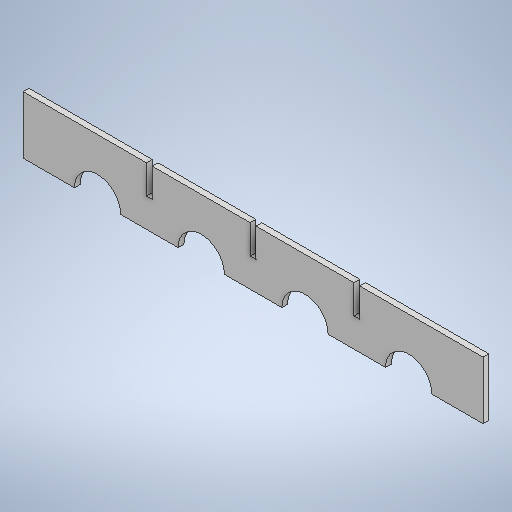
# Autodesk Inventor part: BSH 083 amplifier bottom
Saved by Autodesk Inventor 2025 (Build 290162010, 162A)
## iProperties
Created: 2024-08-04
Part Number: BSH 083 amplifier bottom
Material: Stainless Steel
Document SubType Name: Sheet Metal
Designer: pokla
Density: 8 g/cm^3
Sheet Metal Rule: AISI304 2mm Die16
Appearance: Default
Author: pokla
Autodesk Inventor part; units mm, degrees
ref_plane "YZ Plane" through (0, 0, 0) normal (1, 0, 0) x (0, 1, 0)
ref_plane "XZ Plane" through (0, 0, 0) normal (0, 1, 0) x (-1, 0, 0)
ref_plane "XY Plane" through (0, 0, 0) normal (0, 0, 1) x (1, 0, 0)
sketch "Sketch1" plane through (0, 0, 0) normal (0, 0, 1) x (1, 0, 0)
  circle A0 centre (0, 0) radius 400 construction
  line L0 (-399, 5) -> (399, 5)
  line L1 (399, 5) -> (399, -5)
  line L2 (399, -5) -> (-399, -5)
  line L3 (-399, -5) -> (-399, 5)
  line L4 (-399, 5) -> (399, -5) construction
  dimension "d0" = 800
  dimension "d1" = 10
  dimension "d2" = 798
  constraints: 10 end point, 3 coincident, 2 parallel, 1 centre point, 1 horizontal, 1 midpoint, 1 perpendicular
  measures "d0" diameter of A0
  measures "d1" distance of L0.end L1.end
  measures "d2" distance of L0.start L0.end
extrude "Extrusion1" add sketch "Sketch1" along normal blind 100
sketch "Sketch2" plane through (-399, -5, 0) normal (0, -1, 0) x (1, 0, 0)
  circle A0 centre (309, 0) radius 40
  line L0 (0, 0) -> (798, 0) projected
  circle A1 centre (129, 0) radius 40
  circle A2 centre (489, 0) radius 40
  circle A3 centre (669, 0) radius 40
  line L1 (394, 100) -> (404, 100)
  line L2 (404, 100) -> (404, 50)
  line L3 (404, 50) -> (394, 50)
  line L4 (394, 50) -> (394, 100)
  line L5 (0, 100) -> (798, 100) projected
  line L6 (214, 100) -> (224, 100)
  line L7 (224, 100) -> (224, 50)
  line L8 (224, 50) -> (214, 50)
  line L9 (214, 50) -> (214, 100)
  line L10 (574, 100) -> (584, 100)
  line L11 (584, 100) -> (584, 50)
  line L12 (584, 50) -> (574, 50)
  line L13 (574, 50) -> (574, 100)
  point P0 (399, 0)
  point P1 (399, 0)
  point P2 (399, 0)
  point P3 (399, 0)
  point P4 (399, 100)
  point P5 (219, 100)
  point P6 (399, 100)
  point P7 (399, 100)
  point P8 (579, 100)
  point P9 (399, 100)
  point P10 (399, 100)
  point P11 (709, 0)
  point P12 (629, 0)
  point P13 (529, 0)
  point P14 (449, 0)
  point P15 (269, 0)
  point P16 (349, 0)
  point P17 (169, 0)
  point P18 (89, 0)
  dimension "d5" = 80
  dimension "d7" = 90
  dimension "d8" = 80
  dimension "d9" = 180
  dimension "d10" = 80
  dimension "d11" = 80
  dimension "d12" = 90
  dimension "d13" = 180
  dimension "d14" = 10
  dimension "d15" = 50
  dimension "d16" = 180
  dimension "d17" = 10
  dimension "d18" = 50
  dimension "d19" = 180
  dimension "d20" = 10
  dimension "d21" = 50
  constraints: 24 end point, 8 midpoint, 6 parallel, 4 centre point, 3 horizontal, 3 horizontal alignment, 3 perpendicular, 7 other
  measures "d5" diameter of A0
  measures "d7" distance of point (399, 0) A0.centre
  measures "d8" diameter of A1
  measures "d9" distance of A0.centre A1.centre
  measures "d10" diameter of A2
  measures "d11" diameter of A3
  measures "d12" distance of A2.centre point (399, 0)
  measures "d13" distance of A3.centre A2.centre
  measures "d14" distance between parallel lines of L4 L2
  measures "d15" distance of L3.end L1.start
  measures "d16" distance of point (399, 100) point (219, 100)
  measures "d17" distance between parallel lines of L9 L7
  measures "d18" distance of L8.end L6.start
  measures "d19" distance of point (579, 100) point (399, 100)
  measures "d20" distance between parallel lines of L13 L11
  measures "d21" distance of L12.end L10.start
extrude "Extrusion2" cut sketch "Sketch2" against normal through all contours L0 A0 | L0 A1 | A3 L0 | A2 L0 | L5 L11 L12 L13 | L1 L2 L3 L4 | L7 L8 L9 L5 picked at (302.3333, 20.5179) picked at (130.5738, 20.5179) picked at (658.2131, 7.8371) picked at (497.9217, 9.9086)
equation "\"d17\" = d14"
equation "\"d18\" = d15"
equation "\"d20\" = d14"
equation "\"d21\" = d15"
equation "\"BendReliefWidth\" = Thickness"
equation "\"BendReliefDepth\" = 0.5 * Thickness"
equation "\"CornerReliefSize\" = 4 * Thickness"
equation "\"MinimumRemnant\" = 2 * Thickness"
equation "\"TransitionRadius\" = BendRadius"
equation "\"JacobiRadiusSize\" = BendRadius"
equation "\"GapSize\" = Thickness"
equation "\"Thickness\" = 2"
equation "\"BendRadius\" = 2.75"
body "Solid1"
